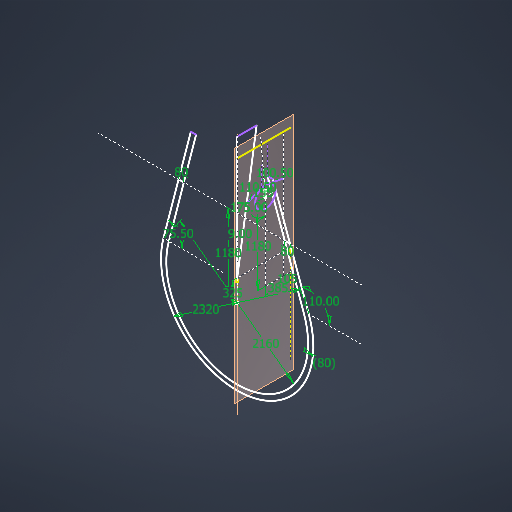
# Autodesk Inventor part: Part1
Saved by Autodesk Inventor 2026.2 (Build 302298000, 298)
## iProperties
Created: 2025-12-11
Part Number: Part1
Material: Generic
Document SubType Name: Modeling
Designer: bubim
Density: 1 g/cm^3
Appearance: Default
Author: bubim
Autodesk Inventor part; units mm, degrees
ref_plane "YZ Plane" through (0, 0, 0) normal (1, 0, 0) x (0, 1, 0)
ref_plane "XZ Plane" through (0, 0, 0) normal (0, 1, 0) x (-1, 0, 0)
ref_plane "XY Plane" through (0, 0, 0) normal (0, 0, 1) x (1, 0, 0)
sketch "Sketch1" plane through (0, 0, 0) normal (0, 0, 1) x (1, 0, 0)
  arc A0 (-1040.2135, 290.4408) -> (1016.915, 363.7084) centre (0, 0) ccw
  arc A1 (-1123.0513, 290.4408) -> (1090.0434, 396.7434) centre (0, 0) ccw
  line L0 (-1123.0513, 290.4408) -> (-892.9956, 1180)
  line L1 (-1123.0513, 290.4408) -> (-204.2253, 290.4408) construction
  line L2 (1090.0434, 396.7434) -> (804.9613, 1180)
  line L3 (1090.0434, 396.7434) -> (1923.5677, 396.7434) construction
  line L4 (0, 0) -> (0, 1180) construction
  line L5 (0, 1180) -> (1900.8085, 1180) construction
  line L6 (1900.8085, 1180) -> (-2124.9709, 1180) construction
  line L7 (804.9613, 1180) -> (724.9613, 1180) construction
  line L8 (804.9613, 1180) -> (724.9613, 1180)
  line L9 (724.9613, 1180) -> (1016.915, 363.7084)
  line L10 (-892.9956, 1180) -> (-812.9956, 1180)
  line L11 (-812.9956, 1180) -> (-1046.3284, 267.5759)
  line L12 (-892.9956, 1180) -> (-706.0774, 1902.7592)
  line L13 (-706.0774, 1902.7592) -> (-626.0774, 1902.7592)
  line L14 (-626.0774, 1902.7592) -> (-812.9956, 1180)
  line L15 (724.9613, 1180) -> (461.8985, 1902.7592)
  line L16 (461.8985, 1902.7592) -> (541.8985, 1902.7592)
  line L17 (541.8985, 1902.7592) -> (804.9613, 1180)
  dimension "d1" = 2160
  dimension "d2" = 2320
  dimension "d4" = 80
  dimension "d5" = 75.5
  dimension "d6" = 110
  dimension "d7" = 1180
  dimension "d8" = 80
  dimension "d9" = 80
  constraints: 36 end point, 6 point on line, 5 point on circle, 4 horizontal, 4 tangent, 3 parallel, 2 centre point, 2 collinear, 2 equal length, 1 coincident, 1 perpendicular, 1 vertical, 1 other
  measures "d1" diameter of A0
  measures "d2" diameter of A1
  measures "d4" radial gap between concentric circles of A1 A0
  measures "d5" angle of L1 L0
  measures "d6" angle of L3 L2
  measures "d7" distance of L4.start L4.end
  measures "d8" distance of L2.end L7.end
  measures "d9" distance of L0.end L10.end
extrude "Extrusion1" add sketch "Sketch1" against normal blind 815
ref_plane "Work Plane1" through (0, 0, 0) normal (1, 0, 0) x (0, 1, 0)
sketch "Sketch2" plane through (0, 0, 0) normal (1, 0, 0) x (0, 1, 0)
  line L0 (0, 0) -> (325, 0) construction
  line L1 (396.7434, 0) -> (-1160, 0) construction
  line L2 (325, 0) -> (325, -815) construction
  line L3 (-1160, -815) -> (396.7434, -815) construction
  line L4 (325, 0) -> (2190.7363, -295.5036)
  line L5 (325, 0) -> (2213.9929, 0) construction
  line L6 (2190.7363, -295.5036) -> (2190.7363, 0)
  line L7 (1902.7592, 0) -> (1902.7592, -815) projected
  line L8 (2190.7363, 0) -> (325, 0)
  line L9 (0, -815) -> (0, -430) construction
  line L10 (0, -430) -> (1180, -430) construction
  line L11 (1180, -430) -> (2009.1519, -357.4586) construction
  line L12 (1180, -430) -> (1334.4102, -416.4909) construction
  arc A0 (1180, -416.4909) -> (1180, -430) centre (1257.2051, -423.2454) ccw
  line L13 (1334.4102, -416.4909) -> (1425.0777, -416.4909) construction
  circle A1 centre (1180, -430) radius 155
  line L14 (1325.1842, -375.7179) -> (1238.8234, -144.7354)
  line L15 (1325.1842, -375.7179) -> (1634.9707, -375.7179) construction
  line L16 (1332.4045, -458.2465) -> (1285.7448, -710)
  line L17 (1332.4045, -458.2465) -> (1864.0398, -458.2465) construction
  line L18 (0, -815) -> (0, -710) construction
  line L19 (0, -710) -> (1902.7592, -710) construction
  point P0 (290.4408, 0)
  point P1 (290.4408, -815)
  dimension "d13" = 325
  dimension "d14" = 9
  dimension "d17" = 385
  dimension "d18" = 1180
  dimension "d19" = 175
  dimension "d20" = 155
  dimension "d22" = 110.5
  dimension "d23" = 100.5
  dimension "d24" = 105
  constraints: 34 end point, 9 point on line, 4 horizontal, 4 perpendicular, 4 point on circle, 2 centre point, 2 coincident, 2 tangent, 1 equal length, 1 midpoint, 1 parallel, 1 vertical, 1 other
  measures "d13" distance of L0.start L0.end
  measures "d14" angle of L4 L5
  measures "d17" distance of L9.start L9.end
  measures "d18" distance of L9.end L10.end
  measures "d19" angle of L11 L10
  measures "d20" distance of L12.end L10.end
  measures "d22" angle of L15 L14
  measures "d23" angle of L16 L17
  measures "d24" distance of L9.start L18.end
extrude "Extrusion2" cut sketch "Sketch2" along normal through all both and the other way through all contours L8 L7 L4 | L8 L6 L4 L7
body "Solid1"
